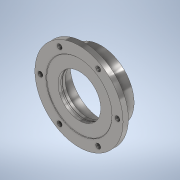
# Autodesk Inventor part: 轴承通盖
Saved by Autodesk Inventor 2020 (Build 240168000, 168)
## iProperties
Created: 2021-06-16
Part Number: 轴承通盖
Material: 常规
Document SubType Name: Modeling
Designer: dell
Density: 1 g/cm^3
Appearance: 默认
Author: dell
Autodesk Inventor part; units mm, degrees
ref_plane "YZ Plane" through (0, 0, 0) normal (1, 0, 0) x (0, 1, 0)
ref_plane "工作平面1" through (0, 0, 0) normal (0, 0, 1) x (1, 0, 0)
sketch "草图1" plane through (0, 0, 0) normal (0, 0, 1) x (1, 0, 0)
  arc A0 (50, 75) -> (50, -75) centre (50, 0) ccw construction
  line L0 (50, 75) -> (50, 100) construction
  arc A1 (50, 100) -> (50, -100) centre (50, 0) ccw construction
  line L1 (50, -100) -> (50, -75) construction
  circle A2 centre (50, 0) radius 100
  circle A3 centre (50, 0) radius 87.5 construction
  line L2 (190.8101, 0) -> (-90.8101, 0) construction
  circle A4 centre (137.5, 0) radius 5.5
  circle A5 centre (93.75, 75.7772) radius 5.5
  circle A6 centre (6.25, 75.7772) radius 5.5
  circle A7 centre (-37.5, 0) radius 5.5
  circle A8 centre (6.25, -75.7772) radius 5.5
  circle A9 centre (93.75, -75.7772) radius 5.5
  point P0 (0, 0)
  dimension "d0" = 175
  dimension "d1" = 11
  dimension "d4" = 360
  constraints: 7 centre point, 3 coincident, 2 end point, 1 concentric, 1 horizontal, 1 horizontal alignment, 1 midpoint, 1 point on line, 15 other
  measures "d1" diameter of A4
extrude "拉伸1" add sketch "草图1" along normal blind 12
sketch "草图2" plane through (50, 0, 12) normal (0, 0, 1) x (1, 0, 0)
  circle A0 centre (0, 0) radius 48 construction
  circle A1 centre (0, 0) radius 48.5
  point P0 (-50, 0)
  dimension "d19" = 97
  constraints: 1 centre point
  measures "d19" diameter of A1
extrude "拉伸2" cut sketch "草图2" against normal up to surface (12 mm away)
sketch "草图3" plane through (50, 0, 0) normal (0, 0, -1) x (-1, 0, 0)
  circle A0 centre (0, 0) radius 100 projected
  circle A1 centre (0, 0) radius 75
  circle A2 centre (0, 0) radius 70
  point P0 (50, 0)
  dimension "d11" = 150
  dimension "d12" = 140
  constraints: 2 centre point, 2 coincident
  measures "d11" diameter of A1
  measures "d12" diameter of A2
extrude "拉伸3" add sketch "草图3" along normal blind 38 contours A1
sketch "草图4" plane through (50, 0, 12) normal (0, 0, 1) x (1, 0, 0)
  circle A0 centre (0, 0) radius 48.5 construction
  circle A1 centre (0, 0) radius 75
  point P0 (-50, 0)
  dimension "d15" = 150
  constraints: 1 centre point, 1 coincident
  measures "d15" diameter of A1
extrude "拉伸4" cut sketch "草图4" against normal blind 1
fillet "圆角1" radius 1 1 edges at (-25, 0, 11)
sketch "草图5" plane through (50, 0, 0) normal (0, 0, -1) x (-1, 0, 0)
  circle A0 centre (0, 0) radius 70 projected
  circle A1 centre (0, 0) radius 48.5 projected
  point P0 (50, 0)
extrude "拉伸5" add sketch "草图5" along normal blind 5
ref_plane "工作平面2" through (50, 0, 3) normal (0, 0, -1) x (-1, 0, 0)
sketch "草图6" plane through (50, 0, 3) normal (0, 0, -1) x (-1, 0, 0)
  circle A0 centre (0, 0) radius 48.5 construction
  circle A1 centre (0, 0) radius 49.275
  point P0 (50, 0)
  dimension "d22" = 98.55
  constraints: 1 centre point, 1 coincident
  measures "d22" diameter of A1
extrude "拉伸6" cut sketch "草图6" against normal mid plane 3.55
sketch "草图7" plane through (50, 0, 0) normal (0, 0, -1) x (-1, 0, 0)
  circle A0 centre (0, 0) radius 48.5 construction
  circle A1 centre (0, 0) radius 75 projected
  circle A2 centre (0, 0) radius 74
  point P0 (50, 0)
  dimension "d25" = 1
  constraints: 1 centre point
  measures "d25" radial gap between concentric circles of A1 A2
extrude "拉伸7" cut sketch "草图7" along normal blind 2
